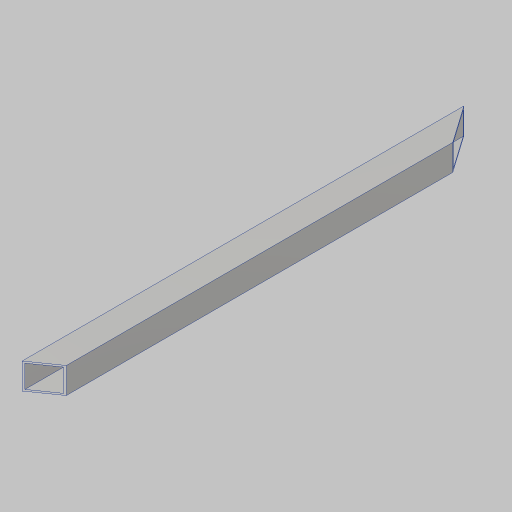
# Autodesk Inventor part: CL-002
Saved by Autodesk Inventor 2023.5 (Build 275446000, 446)
## iProperties
RuleStatus: InUse
Created: 2025-03-17
Part Number: CL-002
Material: Aluminum 6061
Document SubType Name: Modeling
Designer: dlangdon
Mass: 165.254 g
Surface Area: 775.569 cm^2
Volume: 61.205 cm^3
Density: 2.7 g/cm^3
Appearance: Aluminum - Flat
AfterDocNew0: SHOW
AfterDocOpen0: SHOW
Author: dlangdon
Autodesk Inventor part; units mm, degrees
ref_plane "YZ Plane" through (0, 0, 0) normal (1, 0, 0) x (0, 1, 0)
ref_plane "XZ Plane" through (0, 0, 0) normal (0, 1, 0) x (-1, 0, 0)
ref_plane "XY Plane" through (0, 0, 0) normal (0, 0, 1) x (1, 0, 0)
sketch "Sketch1" plane through (0, 0, 0) normal (0, 0, 1) x (1, 0, 0)
  line L0 (-12.7, -12.7) -> (12.7, -12.7)
  line L1 (12.7, -12.7) -> (12.7, 12.7)
  line L2 (12.7, 12.7) -> (-12.7, 12.7)
  line L3 (-12.7, 12.7) -> (-12.7, -12.7)
  line L4 (-12.7, -12.7) -> (12.7, 12.7) construction
  line L5 (12.7, -12.7) -> (-12.7, 12.7) construction
  line L6 (-11.1125, 11.1125) -> (11.1125, 11.1125)
  line L7 (11.1125, 11.1125) -> (11.1125, -11.1125)
  line L8 (11.1125, -11.1125) -> (-11.1125, -11.1125)
  line L9 (-11.1125, -11.1125) -> (-11.1125, 11.1125)
  point P0 (0, 0)
  dimension "width" = 25.4
  dimension "height" = 25.4
  dimension "thickness" = 1.5875
  constraints: 20 end point, 4 parallel, 2 midpoint, 2 perpendicular, 1 horizontal, 3 other
  measures "width" distance of L2.end L1.end
  measures "height" distance of L1.end L0.end
  measures "thickness" distance between parallel lines of L2 L6
extrude "Extrusion1" add sketch "Sketch1" along normal mid plane 431.8
sketch "Sketch3" plane through (-12.7, 12.7, 215.9) normal (0, 1, 0) x (1, 0, 0)
  line L0 (0, 431.8) -> (0, 0) construction
  line L1 (25.4, 0) -> (0, 0) construction
  line L2 (25.4, 431.8) -> (25.4, 0) construction
  line L3 (0, 431.8) -> (25.4, 431.8) construction
  line L4 (0, 0) -> (0, 431.8) construction
  line L5 (0, 0) -> (25.4, 17.7853)
  line L6 (25.4, 431.8) -> (25.4, 0) construction
  line L7 (0, 0) -> (25.4, 0) construction
  line L8 (0, 0) -> (25.4, 0)
  line L9 (25.4, 0) -> (25.4, 17.7853)
  line L10 (0, 431.8) -> (25.4, 395.525)
  line L11 (25.4, 431.8) -> (0, 431.8) construction
  line L12 (0, 431.8) -> (25.4, 431.8)
  line L13 (25.4, 431.8) -> (25.4, 395.525)
  point P0 (12.7, 215.9)
  dimension "d12" = 55
  constraints: 12 end point, 4 point on line, 3 perpendicular, 1 horizontal
  measures "d12" angle of L3 L10
extrude "Extrusion3" cut sketch "Sketch3" against normal through all
body "Solid1"
